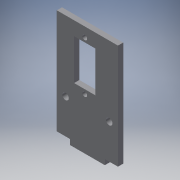
# Autodesk Inventor part: Camera mount raiser
Saved by Autodesk Inventor 2018 (Build 220112000, 112)
## iProperties
Created: 2018-06-25
Part Number: Camera mount raiser
Material: Generic
Document SubType Name: Modeling
Designer: Ajith Thomas
Density: 1 g/cm^3
Appearance: Default
Author: Ajith Thomas
Autodesk Inventor part; units mm, degrees
ref_plane "YZ Plane" through (0, 0, 0) normal (1, 0, 0) x (0, 1, 0)
ref_plane "XZ Plane" through (0, 0, 0) normal (0, 1, 0) x (-1, 0, 0)
ref_plane "XY Plane" through (0, 0, 0) normal (0, 0, 1) x (1, 0, 0)
sketch "Sketch1" plane through (0, 0, 0) normal (0, 0, 1) x (1, 0, 0)
  line L0 (12, 23) -> (0, 23) projected
  line L1 (0, 23) -> (0, 0) projected
  line L2 (0, 0) -> (12, 0) projected
  line L3 (12, 0) -> (12, 23) projected
  line L4 (0, 27.5) -> (5.5, 27.5) construction
  line L5 (6.5, 27.5) -> (12, 27.5) construction
  line L6 (0, -4.5) -> (5.5, -4.5) construction
  line L7 (6.5, -4.5) -> (12, -4.5) construction
  line L8 (-10, 3) -> (-10, 31) construction
  line L9 (25, 31) -> (25, 22) construction
  line L10 (25, 12) -> (25, 3) construction
  circle A0 centre (6, 17) radius 2 construction
  circle A1 centre (6, 17) radius 36.225 construction
  circle A2 centre (6, 17) radius 37.6464 construction
  line L11 (-10, 31) -> (25, 31)
  line L12 (25, 31) -> (25, -29)
  line L13 (25, -29) -> (-10, -29)
  line L14 (-10, -29) -> (-10, 31)
  line L15 (7.5, -29) -> (7.5, 31) construction
  line L16 (-2.5, -29) -> (17.5, -29)
  line L17 (17.5, -29) -> (17.5, -32)
  line L18 (17.5, -32) -> (-2.5, -32)
  line L19 (-2.5, -32) -> (-2.5, -29)
  arc A3 (6.5, -3.804) -> (5.5, -3.804) centre (6, -2.55) ccw construction
  arc A4 (5.5, 26.804) -> (6.5, 26.804) centre (6, 25.55) ccw construction
  circle A5 centre (6, 25.55) radius 1.35
  circle A6 centre (6, -2.55) radius 1.35
  line L20 (12.1, 23.1) -> (-0.1, 23.1)
  line L21 (-0.1, 23.1) -> (-0.1, -0.1)
  line L22 (-0.1, -0.1) -> (12.1, -0.1)
  line L23 (12.1, -0.1) -> (12.1, 23.1)
  point P0 (22, -15.5)
  point P1 (25, -15.5)
  dimension "d0" = 60
  dimension "d1" = 3
  dimension "d2" = 10
  dimension "d3" = 10
  dimension "d4" = 0.1
  dimension "d5" = 0.1
  dimension "d6" = 0.1
  dimension "d7" = 0.1
  constraints: 26 end point, 6 parallel, 4 coincident, 3 horizontal, 3 perpendicular, 2 centre point, 2 concentric, 2 midpoint, 1 point on line, 8 other
  measures "d0" distance of L11.end L12.end
  measures "d1" distance between parallel lines of L16 L18
  measures "d2" distance between parallel lines of L15 L19
  measures "d3" distance between parallel lines of L15 L17
  measures "d4" distance between parallel lines of L0 L20
  measures "d5" distance between parallel lines of L3 L23
  measures "d6" distance between parallel lines of L21 L1
  measures "d7" distance between parallel lines of L2 L22
extrude "Extrusion1" add sketch "Sketch1" along normal blind 3 contours L11 L12 L13 L14 | L13 L17 L18 L19
sketch "Sketch2" plane through (0, 0, 3) normal (0, 0, 1) x (1, 0, 0)
  circle A0 centre (-5, -9.15) radius 1.85 projected
  circle A1 centre (20, -9.15) radius 1.85 projected
  point P0 (0, 0)
extrude "Extrusion2" cut sketch "Sketch2" against normal blind 6.175
body "Solid1"
